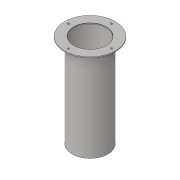
# Autodesk Inventor part: 110mm_flange
Saved by Autodesk Inventor 2016 (Build 200138000, 138)
## iProperties
Created: 2015-09-16
Part Number: 110mm_flange
Material: Generic
Document SubType Name: Modeling
Designer: KA ROSIE
Density: 1 g/cm^3
Appearance: Default
Author: KA ROSIE
Autodesk Inventor part; units mm, degrees
ref_plane "YZ Plane" through (0, 0, 0) normal (1, 0, 0) x (0, 1, 0)
ref_plane "XZ Plane" through (0, 0, 0) normal (0, 1, 0) x (-1, 0, 0)
ref_plane "XY Plane" through (0, 0, 0) normal (0, 0, 1) x (1, 0, 0)
sketch "Sketch1" plane through (0, 0, 0) normal (0, 1, 0) x (-1, 0, 0)
  circle A0 centre (0, 0) radius 52.5
  circle A1 centre (0, 0) radius 82.5
  dimension "d1" = 105
  dimension "d2" = 30
  constraints: 2 centre point, 1 coincident
  measures "d1" diameter of A0
  measures "d2" radial gap between concentric circles of A1 A0
extrude "Extrusion1" add sketch "Sketch1" along normal blind 3
chamfer "Chamfer1" distance 0.5 angle 45 1 edges at (52.5, 3, 0)
sketch "Sketch4" plane through (0, 0, 0) normal (0, -1, 0) x (1, 0, 0)
  circle A0 centre (0, 0) radius 70 construction
  circle A1 centre (0, 70) radius 3
  circle A2 centre (-70, 0) radius 3
  circle A3 centre (0, -70) radius 3
  circle A4 centre (70, 0) radius 3
  dimension "d14" = 140
  dimension "d15" = 6
  dimension "d18" = 360
  constraints: 4 centre point, 1 coincident, 1 vertical alignment, 11 other
  measures "d15" diameter of A1
hole "Hole1" at (0, 0, 70) at (70, 0, 0) at (0, 0, -70) at (-70, 0, 0) direction (0, 1, 0) diameter 6 end through all
sketch "Sketch5" plane through (0, 0, 0) normal (0, -1, 0) x (1, 0, 0)
  circle A0 centre (0, 0) radius 56
  circle A1 centre (0, 0) radius 58
  dimension "d28" = 112
  dimension "d29" = 116
  constraints: 2 centre point, 2 coincident
  measures "d28" diameter of A0
  measures "d29" diameter of A1
extrude "Extrusion3" add sketch "Sketch5" along normal blind 300
body "Solid1"
